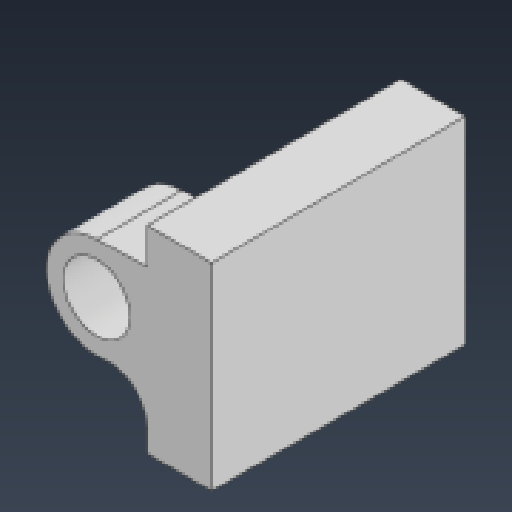
# Autodesk Inventor part: Part15
Saved by Autodesk Inventor 2023 (Build 270158000, 158)
## iProperties
Created: 2025-03-31
Part Number: Part15
Material: Generic
Document SubType Name: Modeling
Designer: szymo
Density: 1 g/cm^3
Appearance: Default
Author: szymo
Autodesk Inventor part; units mm, degrees
ref_plane "YZ Plane" through (0, 0, 0) normal (1, 0, 0) x (0, 1, 0)
ref_plane "XY Plane" through (0, 0, 0) normal (0, 0, 1) x (1, 0, 0)
sketch "Sketch1" plane through (0, 0, 0) normal (0, 0, 1) x (1, 0, 0)
  line L0 (5.7981, 18.3585) -> (13.3674, 18.3585)
  line L1 (13.3674, 18.3585) -> (13.3674, -4.8148)
  line L2 (13.3674, -4.8148) -> (5.7981, -4.8148)
  line L3 (5.7981, -4.8148) -> (5.7981, 18.3585)
  circle A0 centre (-0.1019, 8.0796) radius 2.84 projected
  circle A1 centre (-0.1019, 8.0796) radius 3.9
  circle A2 centre (-0.1019, 8.0796) radius 5.9
  arc A3 (5.7981, -2.2787) -> (0.6626, 2.2293) centre (1.2517, -2.2787) ccw
  line L4 (-0.1019, 13.9796) -> (5.7981, 14.205)
  point P0 (0, 0)
  dimension "d0" = 7.8
  dimension "d1" = 2
  constraints: 10 end point, 4 point on circle, 3 centre point, 3 tangent, 2 parallel, 2 point on line, 1 coincident, 1 horizontal, 1 perpendicular
  measures "d0" diameter of A1
  measures "d1" radial gap between concentric circles of A1 A2
ref_plane "Work Plane1" through (-3.2841, 4.8974, -29.75) normal (0, 0, -1) x (0.075061, 0.9971789, 0)
extrude "Extrusion1" add sketch "Sketch1" against normal up to surface (29.75 mm away) contours L0 L1 L2 L3
sketch "Sketch2" plane through (5.7981, -4.8148, -29.75) normal (-1, 0, 0) x (0, 0, 1)
  line L0 (29.75, 23.1733) -> (0, 23.1733) projected
  line L1 (16.1817, 23.1733) -> (6.6582, 23.1733)
  line L2 (6.6582, 23.1733) -> (6.6582, 6.9688)
  line L3 (6.6582, 6.9688) -> (16.1817, 6.9688)
  line L4 (16.1817, 6.9688) -> (16.1817, 23.1733)
  point P0 (29.75, 4.8148)
  point P1 (6.6582, 23.1733)
  constraints: 8 end point, 2 parallel, 1 horizontal, 1 perpendicular, 1 point on line
extrude "Extrusion3" add sketch "Sketch2" along normal blind 20 separate body
extrude "Extrusion4" add sketch "Sketch1" against normal blind 12.5 contours L3 A2 L4 | A2 | L3 A3 A2 bodies 1
chamfer "Chamfer1" distance 1 distance2 2 1 edges at (-4.0019, 8.0796, -12.5) measured on face at (-4.5019, 8.0796, -12.5)
sketch "Sketch3" plane through (0, 0, 0) normal (0, 1, 0) x (-1, 0, 0)
  line L0 (13.1982, -9.2227) -> (13.1982, -12.9727)
  line L1 (13.1982, -12.9727) -> (8.1982, -12.9727)
  line L2 (8.1982, -12.9727) -> (8.1982, -11.8227)
  line L3 (8.1982, -11.8227) -> (12.1982, -11.8227)
  line L4 (12.1982, -11.8227) -> (12.1982, -9.2227)
  line L5 (12.1982, -9.2227) -> (13.1982, -9.2227)
  line L6 (12.1982, -10.8227) -> (13.1982, -10.8227)
  point P0 (0, 0)
  point P1 (12.6982, -9.2227)
  dimension "d13" = 3.75
  dimension "d14" = 5
  dimension "d15" = 1
  dimension "d17" = 1.6
  dimension "d18" = 2.6
  constraints: 14 end point, 6 perpendicular, 2 point on line, 1 midpoint, 1 vertical
  measures "d13" distance of L0.start L0.end
  measures "d14" distance between parallel lines of L2 L0
  measures "d15" distance between parallel lines of L0 L4
  measures "d17" distance from line of point (12.698, -9.223) L6
  measures "d18" distance between parallel lines of L5 L3
revolve "Revolution1" add sketch "Sketch3" angle 360 about axis through (-12.1982, 0, -9.2227) along (-1, 0, 0) separate body contours L0 L1 L2 L3 L4 L6
chamfer "Chamfer2" distance 0.5 angle 45 3 edges at (-13.1982, 0, -5.4727) (-13.1982, 0, -7.6227) (-8.1982, 0, -6.6227)
ref_plane "Work Plane2" through (-35.7912, -142.2113, -22.4888) normal (-0.9843359, 0.1763032, 0) x (-0.1763032, -0.9843359, 0)
sketch "Sketch4" plane through (-35.7912, -142.2113, -22.4888) normal (-0.9843359, 0.1763032, 0) x (-0.1763032, -0.9843359, 0)
  line L0 (2.8304, -16.6074) -> (4.7198, -9.5562) projected
  line L1 (4.7198, -9.5562) -> (4.0715, -9.3825) projected
  line L2 (4.0715, -9.3825) -> (0.4189, 16.6074) projected
  line L3 (0.4189, 16.6074) -> (-4.7198, 16.6074) projected
  line L4 (-4.7198, 16.6074) -> (-4.7198, -14.5843) projected
  line L5 (-4.7198, -14.5843) -> (2.8304, -16.6074) projected
  line L6 (-11.5025, -6.2926) -> (-11.5025, 5.7074) projected
  line L7 (-11.5025, -6.2926) -> (-4.7198, -6.2926) projected
  line L8 (-4.7198, 5.7074) -> (-4.7198, -6.2926) projected
  line L9 (-4.7198, 5.7074) -> (-11.5025, 5.7074) projected
  line L10 (2.8304, -16.6074) -> (11.5237, -18.9368) projected
  line L11 (11.5237, -18.9368) -> (6.2204, -9.7512) projected
  line L12 (6.2204, -9.7512) -> (4.7716, -9.363) projected
  line L13 (4.7716, -9.363) -> (2.8304, -16.6074) projected
  line L14 (11.5237, -18.9368) -> (-36.6285, -18.9368)
  circle A0 centre (-8.8485, -6.2926) radius 23.9772
  line L15 (11.5237, -18.9368) -> (-1.867, -40.5118)
  line L16 (-1.867, -40.5118) -> (-36.6285, -18.9368)
  point P0 (-146.2938, 22.4888)
  constraints: 6 end point, 1 coincident, 1 horizontal, 1 perpendicular, 1 point on line, 4 other
body "Solid1"
body "Solid2"
body "Solid4"
